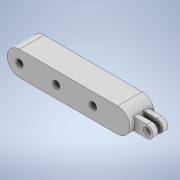
# Autodesk Inventor part: Part7
Saved by Autodesk Inventor 2022 (Build 260153000, 153)
## iProperties
Created: 2022-02-01
Part Number: Part7
Material: Generic
Document SubType Name: Modeling
Designer: br4ch
Density: 1 g/cm^3
Appearance: Default
Author: br4ch
Autodesk Inventor part; units mm, degrees
ref_plane "YZ Plane" through (0, 0, 0) normal (1, 0, 0) x (0, 1, 0)
sketch "Sketch1" plane through (0, 0, 0) normal (0, 0, 1) x (1, 0, 0)
  line L0 (-21.1783, 3) -> (58.8217, 3) construction
  line L1 (-21.1783, -7) -> (58.8217, -7)
  line L2 (58.8217, 13) -> (-21.1783, 13)
  arc A0 (-21.1783, 13) -> (-21.1783, -7) centre (-21.1783, 3) ccw
  arc A1 (58.8217, -7) -> (58.8217, 13) centre (58.8217, 3) ccw
  line L3 (67.482, 8) -> (78.8217, 8)
  arc A2 (78.8217, -2) -> (78.8217, 8) centre (78.8217, 3) ccw
  line L4 (67.482, -2) -> (78.8217, -2)
  circle A3 centre (78.8217, 3) radius 3
  circle A4 centre (8.8217, 3) radius 3
  circle A5 centre (38.8217, 3) radius 3
  circle A6 centre (-21.1783, 3) radius 3
  point P0 (0, 0)
  dimension "d0" = 20
  dimension "d18" = 10
  dimension "d19" = 20
  dimension "d21" = 6
  dimension "d29" = 30
  dimension "d31" = 30
  constraints: 12 end point, 7 centre point, 7 point on circle, 5 tangent, 3 point on line, 2 horizontal, 2 symmetric about line, 1 coincident, 1 equal radius, 1 parallel
  measures "d0" diameter of A1
  measures "d18" diameter of A2
  measures "d19" distance of A2.centre L0.end
  measures "d21" diameter of A3
  measures "d29" distance of A5.centre A4.centre
  measures "d31" distance of A6.centre A4.centre
extrude "Extrusion1" add sketch "Sketch1" along normal blind 20 contours A0 L2 A1 L1
ref_plane "Work Plane5" through (0, 0, 12) normal (0, 0, 1) x (1, 0, 0)
ref_plane "Work Plane4" through (0, 0, 10) normal (0, 0, 1) x (1, 0, 0)
sketch "Sketch4" plane through (0, 0, 12) normal (0, 0, 1) x (1, 0, 0)
  line L0 (67.482, 8) -> (78.8217, 8) projected
  line L1 (67.482, -2) -> (78.8217, -2) projected
  arc A0 (78.8217, -2) -> (78.8217, 8) centre (78.8217, 3) ccw projected
  circle A1 centre (78.8217, 3) radius 3 projected
  arc A2 (58.8217, -7) -> (58.8217, 13) centre (58.8217, 3) ccw projected
  point P0 (0, 0)
extrude "Extrusion4" add sketch "Sketch4" along normal blind 4
ref_plane "Work Plane6" through (0, 0, 10) normal (0, 0, 1) x (1, 0, 0)
mirror "Mirror2" about plane through (0, 0, 10) normal (0, 0, 1) of "Extrusion4"
equation "\"d18\" = R"
equation "\"d21\" = r"
equation "\"d6\" = w"
equation "\"d22\" = 0.2 * w"
equation "\"r\" = 6"
equation "\"d3\" = 6"
equation "\"d5\" = 6"
equation "\"th\" = 5"
equation "\"R\" = 10"
equation "\"w\" = 20"
equation "\"d20\" = 0.1 * w"
equation "\"d25\" = 6"
body "Solid1"
